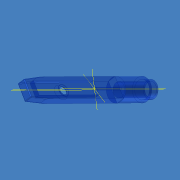
# Autodesk Inventor part: Kopf02
Saved by Autodesk Inventor 2013 (Build 170138000, 138)
## iProperties
Created: 2006-08-08
Part Number: Kopf02
Document SubType Name: Modeling
Designer: acad
Manufacturer: Standard
Standards Organization: Custom
Material: Allgemein
Density: 1 g/cm^3
Author: acad
Autodesk Inventor part; units mm, degrees
ref_plane "YZ Plane" through (0, 0, 0) normal (1, 0, 0) x (0, 1, 0)
ref_plane "XZ Plane" through (0, 0, 0) normal (0, 1, 0) x (-1, 0, 0)
ref_plane "XY Plane" through (0, 0, 0) normal (0, 0, 1) x (1, 0, 0)
sketch "Skizze1" plane through (0, 0, 0) normal (0, 0, 1) x (1, 0, 0)
  line L0 (0, 3.2672) -> (-9, 3.2672)
  line L1 (-9, 3.2672) -> (-9.0128, 3.0688)
  line L2 (-9.0128, 3.0688) -> (-9, 3.2672)
  line L3 (-9, 3.2672) -> (-9, 0.0172)
  line L4 (-9, 0.0172) -> (3, 0.0172)
  line L5 (0, 3.2672) -> (0, 2.5172)
  line L6 (0, 2.5172) -> (3, 2.5172)
  line L7 (3, 2.5172) -> (3, 0.0172)
  dimension "d25" = 3.25
  dimension "d154" = 9
  dimension "d155" = 3
  dimension "d156" = 2.5
  constraints: 17 end point, 2 perpendicular, 1 horizontal, 1 parallel
  measures "d25" distance between parallel lines of L4 L0
  measures "d154" distance of L0.start L0.end
  measures "d155" distance of L5.end L6.end
  measures "d156" distance of L6.end L4.end
revolve "Drehung2" add sketch "Skizze1" angle 360 about axis through (-9, 0.0172, 0) along (1, 0, 0)
sketch "Skizze5" plane through (-9, 0.0172, 0) normal (-1, 0, 0) x (0, 0, 1)
  circle A0 centre (0, 0) radius 3.25 projected
  line L0 (-3, 1.25) -> (-3, -1.25)
  line L1 (-3, -1.25) -> (3, -1.25)
  line L2 (3, -1.25) -> (3, 1.25)
  line L3 (3, 1.25) -> (2, 1.25)
  line L4 (2, 1.25) -> (2, -0.1)
  line L5 (2, -0.1) -> (-2, -0.1)
  line L6 (-2, -0.1) -> (-2, 1.25)
  line L7 (-2, 1.25) -> (-3, 1.25)
  dimension "d63" = 4
  dimension "d66" = 1.15
  dimension "d69" = 2.5
  constraints: 16 end point, 5 parallel, 4 point on circle, 2 perpendicular, 1 collinear, 1 vertical
  measures "d63" distance of L4.end L5.end
  measures "d66" distance between parallel lines of L1 L5
  measures "d69" distance of L0.start L0.end
extrude "Extrusion1" add sketch "Skizze5" along normal blind 31.75 contours L2 L1 L0 L7 L6 L5 L4 L3
chamfer "Fase1" distance 5 distance2 0.5 1 edges at (-40.75, 0.0172, -3) measured on face at (-40.25, 0.0172, -3)
chamfer "Fase2" distance 5 distance2 0.5 1 edges at (-40.75, 0.0172, 3) measured on face at (-40.25, 0.0172, 3)
fillet "Rundung1" radius 0.25 1 edges at (-40.75, 0.0172, -2.5)
fillet "Rundung2" radius 0.25 1 edges at (-40.75, 0.0172, 2.5)
fillet "Rundung3" radius 0.25 5 edges at (-40.75, -1.2328, 0) (-40.6854, -1.2328, -2.4415) (-38.1374, -1.2328, -2.7613) (-40.6854, -1.2328, 2.4415) (-38.1374, -1.2328, 2.7613)
fillet "Rundung4" radius 0.25 6 edges at (-40.75, 1.2672, -2.1369) (-40.6854, 1.2672, -2.4415) (-38.1374, 1.2672, -2.7613) (-40.6854, 1.2672, 2.4415) (-40.75, 1.2672, 2.1369) (-38.1374, 1.2672, 2.7613)
sketch "Skizze11" plane through (-9, 0.0172, 0) normal (-1, 0, 0) x (0, 0, 1)
  line L0 (2, 1.25) -> (3, 1.25) projected
  arc A0 (3, 1.25) -> (-3, 1.25) centre (0, 0) ccw projected
  line L1 (-3, 1.25) -> (-2, 1.25) projected
  line L2 (-2, 1.25) -> (-2, -0.1) projected
  line L3 (-2, -0.1) -> (2, -0.1) projected
  line L4 (2, -0.1) -> (2, 1.25) projected
  line L5 (-2, 1.25) -> (2, 1.25)
  line L6 (2, 1.25) -> (2, -0.1)
  line L7 (2, -0.1) -> (-2, -0.1)
  line L8 (-2, -0.1) -> (-2, 1.25)
  constraints: 8 end point, 2 parallel, 1 horizontal, 1 perpendicular
extrude "Extrusion2" add sketch "Skizze11" along normal blind 8 contours L4 L3 L2 L5
sketch "Skizze18" plane through (-40.75, 0.0172, 0) normal (-1, 0, 0) x (0, 0, 1)
  line L0 (-2, 1) -> (-2, 1.25) projected
  line L1 (-2, 1.25) -> (-2.2738, 1.25) projected
  line L2 (-2.2738, 1.25) -> (-2.2738, 1) projected
  line L3 (-2.2738, 1) -> (-2, 1) projected
  line L4 (2, 1.25) -> (2, 1) projected
  line L5 (2, 1) -> (2.2738, 1) projected
  line L6 (2.2738, 1) -> (2.2738, 1.25) projected
  line L7 (2.2738, 1.25) -> (2, 1.25) projected
  line L8 (-2, 1.25) -> (2, 1.25)
  line L9 (2, 1.25) -> (2, -0.1)
  line L10 (2, -0.1) -> (-2, -0.1)
  line L11 (-2, -0.1) -> (-2, 1.25)
  constraints: 8 end point, 2 parallel, 1 horizontal, 1 perpendicular
extrude "Extrusion3" add sketch "Skizze18" against normal blind 3 contours L0 L8 L4 L9 L10 L11
fillet "Rundung5" radius 0.25 1 edges at (-40.75, 1.2672, 0)
sketch "Skizze19" plane through (-17, -0.0828, 2) normal (0, 1, 0) x (1, 0, 0)
  line L0 (-28.125, 2) -> (33.125, 2) projected
  line L1 (17, -1.25) -> (17, 5.25) projected
  point P0 (-10, 2)
  dimension "d153" = 27
  constraints: 1 point on line
  measures "d153" distance from line of L1 point (-10, 2)
hole "Bohrung11" at (-27, -0.0828, 0) direction (0, -1, 0) diameter 3.2 depth 0.15
sketch "Skizze20" plane through (-9, -1.2328, -3) normal (0, -1, 0) x (1, 0, 0)
  circle A0 centre (-18, 3) radius 1.6 projected
  constraints: 1 coincident
hole "Bohrung12" at (-27, -1.2328, 0) direction (0, 1, 0) diameter 2.2 depth 1 countersink diameter 4 countersink angle 90
sketch "Skizze21" plane through (3, 0.0172, 0) normal (1, 0, 0) x (0, 0, -1)
  circle A0 centre (0, 0) radius 2.5 projected
  constraints: 1 coincident
hole "Bohrung13" at (3, 0.0172, 0) direction (-1, 0, 0) diameter 4 depth 11
sketch "Skizze23" plane through (-8, 0.0172, 0) normal (1, 0, 0) x (0, 0, -1)
  circle A0 centre (0, 0) radius 2 projected
  point P0 (0, 0.575)
  point P1 (0, 0.575)
  constraints: 1 coincident
hole "Bohrung15" at (-8, 0.5922, 0) direction (-1, 0, 0) diameter 0.8 depth 9
